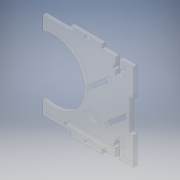
# Autodesk Inventor part: pared frontal 2
Saved by Autodesk Inventor 2016 (Build 200138000, 138)
## iProperties
Created: 2017-02-20
Part Number: pared frontal 2
Material: Generic
Document SubType Name: Modeling
Designer: jorge
Density: 1 g/cm^3
Appearance: Clear - Light
Author: jorge
## iProperties of the stored document pared frontal_3DPrint.ipt
Created: 2017-03-11
Part Number: pared frontal_3DPrint
Material: Generic
Document SubType Name: Modeling
Designer: jorge
Density: 1 g/cm^3
Appearance: Default
Author: jorge
Autodesk Inventor part; units mm, degrees
ref_plane "YZ Plane" through (0, 0, 0) normal (1, 0, 0) x (0, 1, 0)
ref_plane "XZ Plane" through (0, 0, 0) normal (0, 1, 0) x (-1, 0, 0)
ref_plane "XY Plane" through (0, 0, 0) normal (0, 0, 1) x (1, 0, 0)
sketch "Sketch1" plane through (0, 0, 0) normal (0, 0, 1) x (1, 0, 0)
  line L0 (0, 0) -> (25, 0) projected
  line L1 (25, 0) -> (25, 3) projected
  line L2 (0, 3) -> (25, 3) projected
  line L3 (0, 0) -> (0, 3) projected
  line L4 (0.2071, -72) -> (11, -72) projected
  line L5 (0.2071, -69) -> (11, -69) projected
  line L6 (25, -69) -> (50, -69) projected
  line L7 (25, 0) -> (50, 0) projected
  line L8 (-25, 0) -> (0, 0) projected
  line L9 (-22, 0) -> (-22, -10.8146) projected
  line L10 (-25, -22) -> (-25, -47) projected
  line L11 (-25, -47) -> (-22, -47) projected
  line L12 (-22, -10.8146) -> (-22, -58.1854) projected
  line L13 (-25, -22) -> (-22, -22) projected
  line L14 (-22, -58.1854) -> (-22, -69) projected
  line L15 (-25, -69) -> (0, -69) projected
  line L16 (50, 0) -> (50, -22)
  line L17 (50, -22) -> (47, -22)
  line L18 (47, -22) -> (47, -47)
  line L19 (47, -47) -> (50, -47)
  line L20 (50, -47) -> (50, -69)
  line L21 (50, 0) -> (25, 0)
  line L22 (25, 3) -> (25, 0)
  line L23 (25, 3) -> (0, 3)
  line L24 (0, 3) -> (0, 0)
  line L25 (-22, -10.8146) -> (-22, 0)
  line L26 (-22, 0) -> (0, 0)
  line L27 (-22, -22) -> (-25, -22)
  line L28 (-25, -22) -> (-25, -47)
  line L29 (-22, -47) -> (-25, -47)
  line L30 (-22, -58.1854) -> (-22, -69)
  line L31 (-22, -69) -> (0, -69)
  line L32 (0, -72) -> (0, -69)
  line L33 (0, -72) -> (25, -72)
  line L34 (25, -72) -> (25, -69)
  line L35 (25, -69) -> (50, -69)
  line L36 (11, -72) -> (11, -69) projected
  line L37 (0.2071, -69) -> (0.2071, -72) projected
  dimension "d0" = 3
  constraints: 40 end point, 14 perpendicular, 3 collinear, 1 horizontal, 1 parallel, 1 point on line, 1 vertical
  measures "d0" distance of L16.end L17.end
extrude "Extrusion1" add sketch "Sketch1" along normal blind 3
sketch "Sketch2" plane through (0, 0, 3) normal (0, 0, 1) x (1, 0, 0)
  line L0 (-25, -22) -> (-25, -47) projected
  line L1 (-25, -34.5) -> (7, -34.5)
  line L2 (-25, -34.5) -> (-14, -34.5)
  circle A0 centre (-14, -34.5) radius 21
  circle A1 centre (-14, -34.5) radius 25
  point P0 (0, 0)
  dimension "d3" = 32
  dimension "d4" = 11
  dimension "d5" = 4
  constraints: 4 end point, 1 centre point, 1 coincident, 1 horizontal, 1 horizontal alignment, 1 midpoint, 1 point on line, 2 other
  measures "d3" distance of L1.start L1.end
  measures "d4" distance of L1.start L2.end
extrude "Extrusion2" cut sketch "Sketch2" against normal blind 20 contours A0 | A1
sketch "Sketch3" plane through (0, 0, 3) normal (0, 0, 1) x (1, 0, 0)
  line L0 (-1.2929, -65) -> (30.2929, -65) projected
  line L1 (-4.5, -67) -> (-4.5, -65) projected
  line L2 (33.5, -67) -> (33.5, -65) projected
  line L3 (30.6464, -65) -> (33.5, -65) projected
  line L4 (30.6464, -65) -> (30.2929, -65) projected
  line L5 (30.2929, -67) -> (30.6464, -67) projected
  line L6 (33.5, -67) -> (30.6464, -67) projected
  line L7 (30.2929, -67) -> (-1.2929, -67) projected
  arc A0 (-22, -58.1854) -> (-22, -10.8146) centre (-14, -34.5) ccw projected
  line L8 (-22, -58.1854) -> (-22, -69) projected
  line L9 (-22, -69) -> (0, -69) projected
  line L10 (0, -69) -> (0, -72) projected
  line L11 (50, -69) -> (50, -47) projected
  line L12 (50, -47) -> (47, -47) projected
  line L13 (47, -47) -> (47, -22) projected
  line L14 (47, -22) -> (50, -22) projected
  line L15 (50, -22) -> (50, 0) projected
  line L16 (50, 0) -> (25, 0) projected
  line L17 (25, 0) -> (25, 3) projected
  line L18 (25, 3) -> (0, 3) projected
  line L19 (0, 3) -> (0, 0) projected
  line L20 (0, 0) -> (-22, 0) projected
  line L21 (-22, 0) -> (-22, -10.8146) projected
  line L22 (-4.5, -65) -> (-1.6464, -65) projected
  line L23 (-1.2929, -65) -> (-1.6464, -65) projected
  line L24 (-1.6464, -67) -> (-4.5, -67) projected
  line L25 (-1.6464, -67) -> (-1.2929, -67) projected
  line L26 (0, -72) -> (25, -72) projected
  line L27 (25, -69) -> (50, -69) projected
  line L28 (25, -72) -> (25, -69) projected
extrude "Extrusion3" cut sketch "Sketch3" against normal blind 3 contours L0 L4 L3 L2 L6 L5 L7 L25 L24 L1 L22 L23
sketch "Sketch4" plane through (0, 0, 3) normal (0, 0, 1) x (1, 0, 0)
  line L0 (47, -47) -> (47, -22) projected
  line L1 (47, -34.5) -> (34.3, -34.5)
  line L2 (34.3, -34.5) -> (34.3, -36)
  line L3 (34.3, -36) -> (34.3, -33)
  line L4 (34.3, -33) -> (47, -33)
  line L5 (47, -33) -> (47, -36)
  line L6 (47, -36) -> (34.3, -36)
  line L7 (40.65, -36) -> (40.65, -38)
  line L8 (40.65, -38) -> (38.15, -38)
  line L9 (38.15, -38) -> (38.15, -31)
  line L10 (38.15, -31) -> (40.65, -31)
  line L11 (40.65, -31) -> (40.65, -36)
  line L12 (25, 3) -> (0, 3) projected
  line L13 (50, 0) -> (25, 0) projected
  line L14 (0, 0) -> (-22, 0) projected
  line L15 (25, -69) -> (50, -69) projected
  line L16 (0, -72) -> (25, -72) projected
  line L17 (-22, -69) -> (0, -69) projected
  line L18 (50, 0) -> (25, 0) projected
  line L19 (37.5, 0) -> (37.5, -12.7)
  line L20 (37.5, -12.7) -> (39, -12.7)
  line L21 (39, -12.7) -> (36, -12.7)
  line L22 (36, -12.7) -> (36, 0)
  line L23 (39, 0) -> (39, -12.7)
  line L24 (36, -6.35) -> (34, -6.35)
  line L25 (34, -6.35) -> (34, -8.85)
  line L26 (34, -8.85) -> (41, -8.85)
  line L27 (41, -8.85) -> (41, -6.35)
  line L28 (41, -6.35) -> (36, -6.35)
  line L29 (50, -69) -> (25, -69)
  line L30 (37.5, -69) -> (37.5, -56.3)
  line L31 (37.5, -56.3) -> (39, -56.3)
  line L32 (39, -56.3) -> (36, -56.3)
  line L33 (36, -56.3) -> (36, -69)
  line L34 (39, -69) -> (39, -56.3)
  line L35 (36, -62.65) -> (34, -62.65)
  line L36 (34, -62.65) -> (34, -60.15)
  line L37 (34, -60.15) -> (41, -60.15)
  line L38 (41, -60.15) -> (41, -62.65)
  line L39 (41, -62.65) -> (36, -62.65)
  line L40 (-4.5, -65) -> (33.5, -65) projected
  line L41 (33.5, -65) -> (33.5, -67) projected
  line L42 (33.5, -67) -> (-4.5, -67) projected
  line L43 (-4.5, -67) -> (-4.5, -65) projected
  arc A0 (-22, -58.1854) -> (-22, -10.8146) centre (-14, -34.5) ccw projected
  line L44 (-22, -58.1854) -> (-22, -69) projected
  line L45 (-22, -69) -> (0, -69) projected
  line L46 (0, -69) -> (0, -72) projected
  line L47 (0, -72) -> (25, -72) projected
  line L48 (25, -69) -> (50, -69) projected
  line L49 (50, -69) -> (50, -47) projected
  line L50 (50, -47) -> (47, -47) projected
  line L51 (47, -47) -> (47, -22) projected
  line L52 (47, -22) -> (50, -22) projected
  line L53 (50, -22) -> (50, 0) projected
  line L54 (50, 0) -> (25, 0) projected
  line L55 (25, 0) -> (25, 3) projected
  line L56 (25, 3) -> (0, 3) projected
  line L57 (0, 3) -> (0, 0) projected
  line L58 (0, 0) -> (-22, 0) projected
  line L59 (-22, 0) -> (-22, -10.8146) projected
  circle A1 centre (12.5, 1.5) radius 1.5
  line L60 (39, -56.3) -> (36, -56.3)
  line L61 (36, -56.3) -> (36, -69)
  line L62 (36, -69) -> (39, -69)
  line L63 (39, -69) -> (39, -56.3)
  circle A2 centre (12.5, -70.5) radius 1.5
  line L64 (25, -72) -> (25, -69) projected
  arc A3 (42.9741, -36.0257) -> (30.0259, -20.7829) centre (36.5, -28.4043) ccw projected
  line L65 (26.9692, -49.6214) -> (42.9741, -36.0257) projected
  arc A4 (14.0209, -34.3786) -> (26.9692, -49.6214) centre (20.4951, -42) ccw projected
  line L66 (30.0259, -20.7829) -> (14.0209, -34.3786) projected
  dimension "d10" = 12.7
  dimension "d11" = 1.5
  dimension "d12" = 3
  dimension "d13" = 2
  dimension "d14" = 2.5
  dimension "d15" = 7
  dimension "d16" = 12.7
  dimension "d17" = 1.5
  dimension "d18" = 3
  dimension "d19" = 2
  dimension "d20" = 2.5
  dimension "d21" = 7
  dimension "d22" = 3
  dimension "d25" = 3
  constraints: 72 end point, 13 perpendicular, 11 symmetric about line, 10 point on line, 4 midpoint, 3 horizontal, 3 parallel, 3 vertical, 2 centre point
  measures "d10" distance of L1.start L1.end
  measures "d11" distance of L1.end L2.end
  measures "d12" distance of L2.end L3.end
  measures "d13" distance of L7.start L7.end
  measures "d14" distance of L7.end L8.end
  measures "d15" distance of L8.end L9.end
  measures "d16" distance of L19.start L19.end
  measures "d17" distance of L19.end L20.end
  measures "d18" distance of L20.end L21.end
  measures "d19" distance of L24.start L24.end
  measures "d20" distance of L24.end L25.end
  measures "d21" distance of L25.end L26.end
  measures "d22" diameter of A1
  measures "d25" diameter of A2
extrude "Extrusion4" cut sketch "Sketch4" against normal blind 25.4 contours A1 | A2 | L15 L30 L39 L34 | L15 L33 L39 L30 | L39 L30 L37 L34 | L34 L37 L38 L39 | L39 L33 L37 L30 | L37 L30 L31 L34 | L35 L36 L37 L33 | L37 L33 L32 L30 | L23 L28 L19 L13 | L19 L28 L22 L13 | L28 L27 L26 L23 | L23 L26 L19 L28 | L19 L26 L22 L28 | L23 L20 L19 L26 | L22 L26 L25 L24 | L19 L21 L22 L26
sketch "Sketch5" plane through (0, 0, 3) normal (0, 0, 1) x (1, 0, 0)
  line L0 (26.9692, -49.6214) -> (42.9741, -36.0257)
  line L1 (44.9164, -38.3121) -> (28.9114, -51.9078)
  line L2 (42.9741, -36.0257) -> (44.9164, -38.3121)
  line L3 (28.9114, -51.9078) -> (26.9692, -49.6214)
  line L4 (30.0259, -20.7829) -> (14.0209, -34.3786)
  line L5 (12.0787, -32.0922) -> (28.0836, -18.4965)
  line L6 (28.0836, -18.4965) -> (30.0259, -20.7829)
  line L7 (14.0209, -34.3786) -> (12.0787, -32.0922)
  arc A0 (10.5873, -50.4164) -> (19.1404, -54.9292) centre (20.4951, -42) ccw
  line L8 (10.5873, -50.4164) -> (12.8737, -48.4741)
  arc A1 (12.8737, -48.4741) -> (19.1404, -51.9078) centre (20.4951, -42) ccw
  line L9 (19.1404, -51.9078) -> (19.1404, -54.9292)
  point P0 (0, 0)
  constraints: 20 end point, 4 point on circle, 2 centre point, 1 vertical, 25 other
extrude "Extrusion5" cut sketch "Sketch5" against normal blind 25.4
sketch "Sketch6" plane through (0, 3, 3) normal (0, 1, 0) x (1, 0, 0)
  line L0 (12.5, 0) -> (12.5, 3) projected
  line L1 (12.5, 3) -> (0, 3) projected
  line L2 (0, 3) -> (0, 0) projected
  line L3 (12.5, 0) -> (0, 0) projected
  line L4 (25, 0) -> (12.5, 0) projected
  line L5 (25, 3) -> (25, 0) projected
  line L6 (25, 3) -> (12.5, 3) projected
  point P0 (0, 3)
extrude "Extrusion6" add sketch "Sketch6" along normal blind 0.5
sketch "Sketch7" plane through (0, -72, 0) normal (0, -1, 0) x (1, 0, 0)
  line L0 (12.5, 3) -> (12.5, 0) projected
  line L1 (0, 3) -> (12.5, 3) projected
  line L2 (0, 0) -> (0, 3) projected
  line L3 (0, 0) -> (12.5, 0) projected
  line L4 (12.5, 0) -> (25, 0) projected
  line L5 (25, 0) -> (25, 3) projected
  line L6 (12.5, 3) -> (25, 3) projected
extrude "Extrusion7" add sketch "Sketch7" along normal blind 0.5
body "Solid1"
